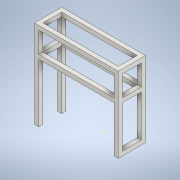
# Autodesk Inventor part: Подлокотник
Saved by Autodesk Inventor 2022 (Build 260153000, 153)
## iProperties
Created: 2021-10-11
Part Number: Подлокотник
Material: Типовые
Document SubType Name: Modeling
Designer: Admin
Density: 1 g/cm^3
Appearance: Сталь
Author: Admin
Autodesk Inventor part; units mm, degrees
ref_plane "YZ Plane" through (0, 0, 0) normal (1, 0, 0) x (0, 1, 0)
ref_plane "XZ Plane" through (0, 0, 0) normal (0, 1, 0) x (-1, 0, 0)
ref_plane "XY Plane" through (0, 0, 0) normal (0, 0, 1) x (1, 0, 0)
sketch "Эскиз1" plane through (0, 0, 0) normal (0, 1, 0) x (-1, 0, 0)
  line L0 (-200, 65) -> (200, 65) construction
  line L1 (200, 65) -> (200, -65) construction
  line L2 (200, -65) -> (-200, -65) construction
  line L3 (-200, -65) -> (-200, 65) construction
  line L4 (-200, 65) -> (200, -65) construction
  line L5 (200, 65) -> (-200, -65) construction
  line L6 (200, 65) -> (180, 65)
  line L7 (180, 65) -> (180, 45)
  line L8 (180, 45) -> (200, 45)
  line L9 (200, 45) -> (200, 65)
  line L10 (200, -65) -> (180, -65)
  line L11 (180, -65) -> (180, -45)
  line L12 (180, -45) -> (200, -45)
  line L13 (200, -45) -> (200, -65)
  line L14 (-200, 65) -> (-180, 65)
  line L15 (-180, 65) -> (-180, 45)
  line L16 (-180, 45) -> (-200, 45)
  line L17 (-200, 45) -> (-200, 65)
  line L18 (-200, -65) -> (-180, -65)
  line L19 (-180, -65) -> (-180, -45)
  line L20 (-180, -45) -> (-200, -45)
  line L21 (-200, -45) -> (-200, -65)
  point P0 (0, 0)
  dimension "d0" = 400
  dimension "d1" = 130
  dimension "d2" = 20
  dimension "d3" = 20
  dimension "d4" = 20
  dimension "d5" = 20
  dimension "d6" = 20
  dimension "d7" = 20
  dimension "d8" = 20
  dimension "d9" = 20
  constraints: 44 end point, 10 parallel, 5 horizontal, 5 perpendicular, 2 midpoint
  measures "d0" distance of L1.end L2.end
  measures "d1" distance of L0.end L1.end
  measures "d2" distance of L8.end L7.end
  measures "d3" distance of L7.end L6.end
  measures "d4" distance of L11.end L12.end
  measures "d5" distance of L10.end L11.end
  measures "d6" distance of L15.end L16.end
  measures "d7" distance of L14.end L15.end
  measures "d8" distance of L20.end L19.end
  measures "d9" distance of L19.end L18.end
extrude "Выдавливание1" add sketch "Эскиз1" along normal blind 400
sketch "Эскиз2" plane through (200, 0, 65) normal (1, 0, 0) x (0, 0, -1)
  line L0 (20, 400) -> (0, 400) projected
  line L1 (0, 400) -> (20, 400)
  line L2 (20, 400) -> (20, 420)
  line L3 (20, 420) -> (0, 420)
  line L4 (0, 420) -> (0, 400)
  line L5 (130, 0) -> (130, 400) projected
  line L6 (130, 400) -> (110, 400)
  line L7 (110, 400) -> (110, 420)
  line L8 (110, 420) -> (130, 420)
  line L9 (130, 420) -> (130, 400)
  line L10 (0, 0) -> (0, 400) projected
  line L11 (0, 280) -> (20, 280)
  line L12 (20, 280) -> (20, 300)
  line L13 (20, 300) -> (0, 300)
  line L14 (0, 300) -> (0, 280)
  line L15 (110, 300) -> (130, 300)
  line L16 (130, 300) -> (130, 280)
  line L17 (130, 280) -> (110, 280)
  line L18 (110, 280) -> (110, 300)
  point P0 (65, 0)
  point P1 (0, 300)
  dimension "d12" = 20
  dimension "d13" = 20
  dimension "d14" = 20
  dimension "d15" = 20
  dimension "d25" = 20
  dimension "d26" = 20
  dimension "d27" = 100
  dimension "d28" = 20
  dimension "d29" = 20
  dimension "d30" = 100
  dimension "d31" = 90
  constraints: 32 end point, 8 parallel, 4 horizontal, 4 perpendicular, 1 point on line
  measures "d12" distance of L3.end L2.end
  measures "d13" distance of L2.end L1.end
  measures "d14" distance of L7.end L8.end
  measures "d15" distance of L6.end L7.end
  measures "d25" distance of L13.end L12.end
  measures "d26" distance of L12.end L11.end
  measures "d27" distance between parallel lines of L13 L0
  measures "d28" distance of L16.end L17.end
  measures "d29" distance of L15.end L16.end
  measures "d30" distance from line of L5.end L15
  measures "d31" distance between parallel lines of L18 L12
extrude "Выдавливание2" add sketch "Эскиз2" against normal blind 400
sketch "Эскиз3" plane through (-200, 420, 65) normal (0, 0, 1) x (1, 0, 0)
  line L0 (0, -420) -> (0, 0) projected
  line L1 (20, -420) -> (20, -20) projected
  line L2 (0, 0) -> (20, 0)
  line L3 (20, 0) -> (20, -20)
  line L4 (20, -20) -> (0, -20)
  line L5 (0, -20) -> (0, 0)
  line L6 (380, -420) -> (380, -20) projected
  line L7 (400, -420) -> (400, 0) projected
  line L8 (380, -20) -> (400, -20)
  line L9 (400, -20) -> (400, 0)
  line L10 (400, 0) -> (380, 0)
  line L11 (380, 0) -> (380, -20)
  line L12 (0, -140) -> (20, -140)
  line L13 (20, -140) -> (20, -120)
  line L14 (20, -120) -> (0, -120)
  line L15 (0, -120) -> (0, -140)
  line L16 (380, -420) -> (380, -20) projected
  line L17 (400, -420) -> (400, 0) projected
  line L18 (380, -140) -> (400, -140)
  line L19 (400, -140) -> (400, -120)
  line L20 (400, -120) -> (380, -120)
  line L21 (380, -120) -> (380, -140)
  point P0 (200, -420)
  point P1 (20, -120)
  point P2 (0, -120)
  point P3 (20, -140)
  dimension "d20" = 20
  dimension "d21" = 20
  dimension "d22" = 100
  dimension "d23" = 100
  dimension "d24" = 20
  constraints: 32 end point, 8 parallel, 4 horizontal, 4 perpendicular, 3 point on line
  measures "d20" distance of L14.end L13.end
  measures "d21" distance of L13.end L12.end
  measures "d22" distance between parallel lines of L14 L4
  measures "d23" distance between parallel lines of L8 L20
  measures "d24" distance between parallel lines of L18 L20
extrude "Выдавливание3" add sketch "Эскиз3" against normal blind 130 contours L0 L14 L1 L12 | L0 L2 L3 L4 | L6 L20 L7 L18 | L11 L10 L7 L8
sketch "Эскиз4" plane through (200, 420, -65) normal (0, 0, -1) x (-1, 0, 0)
  point P0 (200, -420)
sketch "Эскиз7" plane through (0, 0, 0) normal (0, -1, 0) x (1, 0, 0)
  line L0 (232.9472, 106.3053) -> (134.9615, 106.3053)
  line L1 (134.9615, 106.3053) -> (134.9615, -101.9914)
  line L2 (134.9615, -101.9914) -> (232.9472, -101.9914)
  line L3 (232.9472, -101.9914) -> (232.9472, 106.3053)
  point P0 (0, 0)
  constraints: 8 end point, 2 parallel, 1 horizontal, 1 perpendicular
extrude "Выдавливание5" cut sketch "Эскиз7" against normal blind 80
sketch "Эскиз9" plane through (0, 0, 0) normal (0, 0, 1) x (1, 0, 0)
  line L0 (200, 80) -> (180, 80) projected
  line L1 (200, 80) -> (180, 80)
  line L2 (180, 80) -> (180, 60)
  line L3 (180, 60) -> (200, 60)
  line L4 (200, 60) -> (200, 80)
  point P0 (0, 0)
  dimension "d45" = 20
  dimension "d46" = 20
  constraints: 8 end point, 2 parallel, 1 horizontal, 1 perpendicular
  measures "d45" distance of L3.end L2.end
  measures "d46" distance of L2.end L1.end
extrude "Выдавливание6" add sketch "Эскиз9" along normal mid plane 130
sketch "Эскиз11" plane through (180, 60, 65) normal (0, -1, 0) x (1, 0, 0)
  line L0 (0, -20) -> (20, -20) projected
  line L1 (20, -110) -> (0, -110) projected
  point P0 (-180, -65)
  point P1 (10, -20)
  point P2 (10, -110)
  constraints: 2 midpoint
hole "Отверстие3" at (190, 60, 45) at (190, 60, -45) direction (0, 1, 0) diameter 5 depth 5
